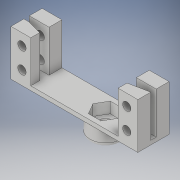
# Autodesk Inventor part: exp0
Saved by Autodesk Inventor 2019 (Build 230136000, 136)
## iProperties
Created: 2019-10-01
Part Number: exp0
Material: Générique
Document SubType Name: Modeling
Designer: dubicube
Density: 1 g/cm^3
Appearance: Par défaut
Author: dubicube
Autodesk Inventor part; units mm, degrees
ref_plane "YZ Plane" through (0, 0, 0) normal (1, 0, 0) x (0, 1, 0)
ref_plane "XZ Plane" through (0, 0, 0) normal (0, 1, 0) x (-1, 0, 0)
ref_plane "XY Plane" through (0, 0, 0) normal (0, 0, 1) x (1, 0, 0)
sketch "Esquisse1" plane through (0, 0, 0) normal (0, 1, 0) x (-1, 0, 0)
  line L0 (0, 0) -> (-61, 0)
  line L1 (-61, 0) -> (-61, -15)
  line L2 (-61, -15) -> (0, -15)
  line L3 (0, -15) -> (0, 0)
  dimension "d0" = 15
  dimension "d1" = 61
  constraints: 8 end point, 2 parallel, 1 horizontal, 1 perpendicular
  measures "d0" distance of L2.end L0.start
  measures "d1" distance of L1.end L2.end
extrude "Extrusion1" add sketch "Esquisse1" along normal blind 2
sketch "Esquisse2" plane through (0, 2, 0) normal (0, 1, 0) x (1, 0, 0)
  line L0 (0, 15) -> (0, 0) projected
  line L1 (0, 0) -> (9.5, 0)
  line L2 (9.5, 0) -> (9.5, 4.3)
  line L3 (0, 6.2) -> (0, 0)
  line L4 (0, 15) -> (9.5, 15)
  line L5 (9.5, 15) -> (9.5, 8.8)
  line L6 (9.5, 8.8) -> (0, 8.8)
  line L7 (0, 8.8) -> (0, 15)
  line L8 (0, 0) -> (61, 0) construction
  line L9 (30.5, 0) -> (30.5, 15) construction
  line L10 (61, 15) -> (61, 0)
  line L11 (61, 0) -> (51.5, 0)
  line L12 (51.5, 0) -> (51.5, 4.3)
  line L13 (51.5, 4.3) -> (61, 6.2)
  line L14 (61, 6.2) -> (61, 0)
  line L15 (61, 15) -> (51.5, 15)
  line L16 (51.5, 15) -> (51.5, 8.8)
  line L17 (51.5, 8.8) -> (61, 8.8)
  line L18 (61, 8.8) -> (61, 15)
  line L19 (0, 6.2) -> (2.5, 6.2)
  line L20 (2.5, 6.2) -> (9.5, 4.3)
  dimension "d33" = 2.6
  dimension "d34" = 6.2
  dimension "d36" = 4.5
  dimension "d37" = 2.5
  dimension "d38" = 7
  constraints: 38 end point, 7 symmetric about line, 3 horizontal, 3 parallel, 2 perpendicular, 1 collinear, 1 midpoint, 1 vertical
  measures "d33" distance of L3.start L6.end
  measures "d34" distance of L4.end L5.end
  measures "d36" distance of L2.end L5.end
  measures "d37" distance of L3.start L19.end
  measures "d38" distance from line of L19.end L2
extrude "Extrusion2" add sketch "Esquisse2" along normal blind 20
sketch "Esquisse3" plane through (0, 0, 0) normal (0, 0, 1) x (1, 0, 0)
  circle A0 centre (55.7, 16.5) radius 2
  line L0 (51.5, 2) -> (51.5, 22) projected
  circle A1 centre (55.7, 6.5) radius 2
  line L1 (51.5, 22) -> (61, 22) projected
  line L2 (0, 0) -> (61, 0) projected
  line L3 (51.5, 2) -> (9.5, 2) construction
  line L4 (30.5, 0) -> (30.5, 2) construction
  line L5 (9.5, 2) -> (51.5, 2) construction
  circle A2 centre (5.3, 16.5) radius 2
  circle A3 centre (5.3, 6.5) radius 2
  dimension "d10" = 4
  dimension "d11" = 4.2
  dimension "d12" = 4.2
  dimension "d40" = 10
  dimension "d41" = 4.5
  constraints: 4 centre point, 2 end point, 2 midpoint, 2 symmetric about line, 1 equal radius, 2 other
  measures "d10" diameter of A0
  measures "d11" distance from line of L0 A0.centre
  measures "d12" distance from line of L0 A1.centre
  measures "d40" distance of A1.centre A0.centre
  measures "d41" distance from line of L3 A1.centre
extrude "Extrusion3" cut sketch "Esquisse3" against normal blind 20
sketch "Esquisse4" plane through (0, 0, 0) normal (0, -1, 0) x (1, 0, 0)
  circle A0 centre (44, -7.5) radius 5.15
  circle A1 centre (44, -7.5) radius 3.15
  line L0 (61, -6.2) -> (61, -8.8) construction
  line L1 (0, -8.8) -> (0, -6.2) construction
  line L2 (0, -15) -> (0, 0) construction
  line L3 (0, 0) -> (61, 0) construction
  line L4 (9.5, 0) -> (51.5, 0) construction
  line L5 (44, 0) -> (44, -15) construction
  line L6 (61, 0) -> (61, -15) construction
  line L7 (61, -15) -> (0, -15) construction
  dimension "d18" = 6.3
  dimension "d19" = 2
  dimension "d21" = 17
  constraints: 2 centre point, 2 coincident, 2 end point, 2 point on line, 1 midpoint, 1 vertical
  measures "d18" diameter of A1
  measures "d19" radial gap between concentric circles of A0 A1
  measures "d21" distance between parallel lines of L6 L5
sketch "Esquisse5" plane through (0, 2, 0) normal (0, 1, 0) x (1, 0, 0)
  circle A0 centre (38, 7.5) radius 3.15 projected
  line L0 (41.0311, 2.25) -> (34.9689, 2.25)
  line L1 (34.9689, 2.25) -> (31.9378, 7.5)
  line L2 (31.9378, 7.5) -> (34.9689, 12.75)
  line L3 (34.9689, 12.75) -> (41.0311, 12.75)
  line L4 (41.0311, 12.75) -> (44.0622, 7.5)
  line L5 (44.0622, 7.5) -> (41.0311, 2.25)
  line L6 (9.5, 0) -> (51.5, 0) projected
  point P0 (0, 0)
  dimension "d24" = 10.5
  constraints: 12 end point, 2 coincident, 1 parallel, 13 other
  measures "d24" distance between parallel lines of L1 L4
sketch "Esquisse7" plane through (0, 0, 0) normal (0, -1, 0) x (1, 0, 0)
  circle A0 centre (38, -7.5) radius 3.15 projected
  circle A1 centre (38, -7.5) radius 7.5
  line L0 (61, -15) -> (0, -15) projected
  point P0 (0, 0)
  constraints: 1 centre point, 1 coincident, 1 tangent
extrude "Extrusion6" add sketch "Esquisse7" along normal blind 8
extrude "Extrusion7" cut sketch "Esquisse5" against normal blind 5.3 contours A0 | L0 L1 L2 L3 L4 L5
fillet "Congé1" radius 2 1 edges at (30.5, -8, -7.5)
equation "\"d12\" = d11"
